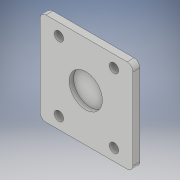
# Autodesk Inventor part: back plate
Saved by Autodesk Inventor 2018 (Build 220112000, 112)
## iProperties
Created: 2018-04-27
Part Number: back plate
Material: Generic
Document SubType Name: Modeling
Designer: 232963
Density: 1 g/cm^3
Appearance: Default
Author: 232963
Autodesk Inventor part; units mm, degrees
ref_plane "YZ Plane" through (0, 0, 0) normal (1, 0, 0) x (0, 1, 0)
ref_plane "XZ Plane" through (0, 0, 0) normal (0, 1, 0) x (-1, 0, 0)
ref_plane "XY Plane" through (0, 0, 0) normal (0, 0, 1) x (1, 0, 0)
sketch "Sketch1" plane through (0, 0, 0) normal (0, 0, 1) x (1, 0, 0)
  line L0 (-19.4132, 28.9616) -> (25.0368, 28.9616)
  line L1 (28.2118, 25.7866) -> (28.2118, -18.6634)
  line L2 (25.0368, -21.8384) -> (-19.4132, -21.8384)
  line L3 (-22.5882, -18.6634) -> (-22.5882, 25.7866)
  circle A0 centre (-12.2504, 22.4846) radius 2.54
  circle A1 centre (17.874, 22.4846) radius 2.54
  circle A2 centre (17.874, -15.3614) radius 2.54
  circle A3 centre (-12.2504, -15.3614) radius 2.54
  arc A4 (-19.4132, 28.9616) -> (-22.5882, 25.7866) centre (-19.4132, 25.7866) ccw
  arc A5 (28.2118, 25.7866) -> (25.0368, 28.9616) centre (25.0368, 25.7866) ccw
  arc A6 (25.0368, -21.8384) -> (28.2118, -18.6634) centre (25.0368, -18.6634) ccw
  arc A7 (-22.5882, -18.6634) -> (-19.4132, -21.8384) centre (-19.4132, -18.6634) ccw
  point P0 (0, 0)
  point P1 (28.2118, -21.8384)
  point P2 (28.2118, 28.9616)
  point P3 (-22.5882, -21.8384)
  dimension "d0" = 50.8
  dimension "d1" = 50.8
  dimension "d2" = 5.08
  dimension "d3" = 5.08
  dimension "d4" = 5.08
  dimension "d5" = 5.08
  dimension "d6" = 37.846
  dimension "d9" = 30.1244
  dimension "d10" = 30.1244
  dimension "d11" = 10.3378
  dimension "d12" = 10.3378
  dimension "d13" = 37.846
  dimension "d14" = 6.477
  dimension "d15" = 6.477
  dimension "d16" = 6.477
  dimension "d17" = 6.477
  dimension "d18" = 3.175
  constraints: 8 centre point, 8 end point, 8 point on circle, 8 tangent, 6 point on line, 3 equal radius, 2 parallel, 1 horizontal, 1 perpendicular
  measures "d0" distance of point (28.212, -21.838) point (-22.588, -21.838)
  measures "d1" distance of point (28.212, 28.962) point (28.212, -21.838)
  measures "d2" diameter of A0
  measures "d3" diameter of A1
  measures "d4" diameter of A2
  measures "d5" diameter of A3
  measures "d6" distance of A3.centre A0.centre
  measures "d9" distance of A1.centre A0.centre
  measures "d10" distance of A2.centre A3.centre
  measures "d11" distance from line of L3 A0.centre
  measures "d12" distance from line of L3 A3.centre
  measures "d13" distance of A2.centre A1.centre
  measures "d14" distance from line of L2 A3.centre
  measures "d15" distance from line of L2 A2.centre
  measures "d16" distance from line of L0 A1.centre
  measures "d17" distance from line of L0 A0.centre
  measures "d18" radius of A4
extrude "Extrusion1" add sketch "Sketch1" along normal blind 3.81
sketch "Sketch2" plane through (0, 0, 3.81) normal (0, 0, 1) x (1, 0, 0)
  circle A0 centre (2.4073, 3.9993) radius 9.0805
  point P0 (0, 0)
  dimension "d21" = 18.161
  constraints: 1 centre point
  measures "d21" diameter of A0
extrude "Extrusion2" cut sketch "Sketch2" against normal blind 2.4384
body "Solid1"
